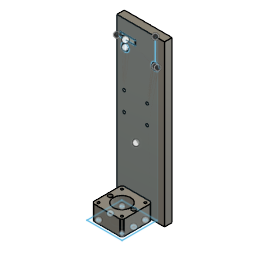
lh_arm_mount_i1 (Autodesk Fusion 360 design; units mm, degrees)
Autodesk Fusion 360 part; units mm, degrees
note: some values were not read from the file. Chosen so that the rebuilt part matches the saved one: which pieces of a blend or face edit are solid.
imported_body "Base Feature1" makes body 1 makes body 2 makes body 3
sketch "Sketch3" plane through (0, 15.85, 0) normal (0, 1, 0) x (-1, 0, 0)
  line L0 (19.8321, 18.0037) -> (18.0037, 19.8321)
  arc A0 (18.0037, 19.8321) -> (17.2966, 20.125) centre (17.2966, 19.125) ccw
  line L1 (17.2966, 20.125) -> (-17.2966, 20.125)
  arc A1 (-17.2966, 20.125) -> (-18.0037, 19.8321) centre (-17.2966, 19.125) ccw
  line L2 (-18.0037, 19.8321) -> (-19.8321, 18.0037)
  arc A2 (-19.8321, 18.0037) -> (-20.125, 17.2966) centre (-19.125, 17.2966) ccw
  line L3 (-20.125, 17.2966) -> (-20.125, -17.2966)
  arc A3 (-20.125, -17.2966) -> (-19.8321, -18.0037) centre (-19.125, -17.2966) ccw
  line L4 (-19.8321, -18.0037) -> (-18.0037, -19.8321)
  arc A4 (-18.0037, -19.8321) -> (-17.2966, -20.125) centre (-17.2966, -19.125) ccw
  line L5 (-17.2966, -20.125) -> (17.2966, -20.125)
  arc A5 (17.2966, -20.125) -> (18.0037, -19.8321) centre (17.2966, -19.125) ccw
  line L6 (18.0037, -19.8321) -> (19.8321, -18.0037)
  arc A6 (19.8321, -18.0037) -> (20.125, -17.2966) centre (19.125, -17.2966) ccw
  line L7 (20.125, -17.2966) -> (20.125, 17.2966)
  arc A7 (20.125, 17.2966) -> (19.8321, 18.0037) centre (19.125, 17.2966) ccw
  circle A8 centre (0, 0) radius 11.5
  line L8 (22.9904, -22.6956) -> (-23.4325, -22.6956)
  line L9 (-23.4325, -22.6956) -> (-23.4325, 23.3044)
  line L10 (-23.4325, 23.3044) -> (22.9904, 23.3044)
  line L11 (22.9904, 23.3044) -> (22.9904, -22.6956)
  circle A9 centre (15.5, 0) radius 2.7
  circle A10 centre (-15.5, 0) radius 2.7
  circle A11 centre (-15.5, 15.5) radius 1.5
  circle A12 centre (15.5, 15.5) radius 1.5
  circle A13 centre (15.5, -15.5) radius 1.5
  circle A14 centre (-15.5, -15.5) radius 1.5
  dimension "d12" = 46
  dimension "d27" = 5.4
  dimension "d28" = 5.4
  dimension "d34" = 3
  dimension "d35" = 3
  dimension "d36" = 3
  dimension "d37" = 3
  constraint horizontal L8
  constraint vertical L9
  constraint horizontal L10
  constraint vertical L11
  measures "d12" distance of L8.start L10.end
  measures "d27" diameter of A9
  measures "d28" diameter of A10
  measures "d34" diameter of A11
  measures "d35" diameter of A12
  measures "d36" diameter of A13
  measures "d37" diameter of A14
extrude "Extrude6" add sketch "Sketch3" along normal blind 20 separate body contours L0 A0 L1 A1 L2 A2 L3 A3 L4 A4 L5 A5 L6 A6 L7 A7 makes body 4
sketch "Sketch5" plane through (0, 0, -20.125) normal (0, 0, -1) x (-1, 0, 0)
  line L0 (-17.2966, 15.85) -> (17.2966, 15.85)
  line L1 (17.2966, 35.85) -> (-17.2966, 35.85)
  line L2 (-27, 227.85) -> (27, 227.85)
  line L3 (27, 227.85) -> (27, 15.85)
  line L4 (27, 15.85) -> (-27, 15.85)
  line L5 (-27, 15.85) -> (-27, 227.85)
  point P0 (0, 15.85)
  dimension "d40" = 54
  dimension "d41" = 212
  constraint horizontal L2
  constraint vertical L3
  constraint horizontal L4
  constraint vertical L5
  constraint midpoint L4 P0
  measures "d40" distance of L2.start L2.end
  measures "d41" distance of L2.start L4.end
extrude "Extrude7" add sketch "Sketch5" along normal blind 10 bodies 4
sketch "Sketch7" plane through (0, 0, -20.125) normal (0, 0, 1) x (1, 0, 0)
  line L0 (17.2966, 35.85) -> (17.2966, 15.85)
  line L1 (17.2966, 15.85) -> (27, 15.85)
  line L2 (27, 15.85) -> (27, 227.85)
  line L3 (27, 227.85) -> (-27, 227.85)
  line L4 (-27, 227.85) -> (-27, 15.85)
  line L5 (-27, 15.85) -> (-17.2966, 15.85)
  line L6 (-17.2966, 15.85) -> (-17.2966, 35.85)
  line L7 (-17.2966, 35.85) -> (17.2966, 35.85)
  line L8 (-17.2966, 35.85) -> (-17.2966, 120.85)
  line L9 (17.2966, 35.85) -> (17.2966, 120.85)
  line L10 (27, 120.85) -> (13.1, 120.85)
  circle A0 centre (13.1, 120.85) radius 1.7
  circle A1 centre (-17.2966, 120.85) radius 1.7
  line L11 (13.1, 120.85) -> (13.1, 145.85)
  line L12 (-17.2966, 120.85) -> (-17.2966, 145.85)
  circle A2 centre (13.1, 145.85) radius 1.7
  circle A3 centre (-17.2966, 145.85) radius 1.7
  dimension "d46" = 85
  dimension "d50" = 85
  dimension "d51" = 13.9
  dimension "d52" = 3.4
  dimension "d54" = 3.4
  dimension "d56" = 25
  dimension "d57" = 25
  dimension "d58" = 3.4
  dimension "d59" = 3.4
  constraint coincident L6.end L7.start
  constraint perpendicular L7 L8
  constraint coincident L0.start L7.end
  constraint perpendicular L7 L9
  constraint coincident L2 L10.start
  constraint perpendicular L2 L10
  constraint coincident L10.end A0.centre
  constraint coincident L8.end A1.centre
  constraint perpendicular L10 L11
  constraint parallel L8 L12
  constraint coincident L11.end A2.centre
  constraint coincident L12.end A3.centre
  measures "d46" distance of L6.end L8.end
  measures "d50" distance of L0.start L9.end
  measures "d51" distance of L10.start L10.end
  measures "d52" diameter of A0
  measures "d54" diameter of A1
  measures "d56" distance of L10.end L11.end
  measures "d57" distance of L8.end L12.end
  measures "d58" diameter of A2
  measures "d59" diameter of A3
hole "Hole2" at (13.1, 120.85, -20.125) at (13.1, 145.85, -20.125) at (-17.2966, 120.85, -20.125) at (-17.2966, 145.85, -20.125) direction (0, 0, -1) diameter 3.4 end through all bodies 4
sketch "Sketch8" plane through (0, 0, -20.125) normal (0, 0, 1) x (1, 0, 0)
  circle A0 centre (-17.2966, 120.85) radius 1.7
  circle A1 centre (13.1, 120.85) radius 1.7
  circle A2 centre (13.1, 145.85) radius 1.7
  circle A3 centre (-17.2966, 145.85) radius 1.7
  line L0 (17.2966, 35.85) -> (17.2966, 15.85)
  line L1 (17.2966, 15.85) -> (27, 15.85)
  line L2 (27, 15.85) -> (27, 227.85)
  line L3 (27, 227.85) -> (-27, 227.85)
  line L4 (-27, 227.85) -> (-27, 15.85)
  line L5 (-27, 15.85) -> (-17.2966, 15.85)
  line L6 (-17.2966, 15.85) -> (-17.2966, 35.85)
  line L7 (-17.2966, 35.85) -> (17.2966, 35.85)
  circle A4 centre (24, 193.8202) radius 4.9
  circle A5 centre (-15.7, 195.8051) radius 4.9
  line L8 (-15.5849, 190.9065) -> (-15.5849, 204.5065)
  line L9 (-27, 204.488) -> (-22, 204.488)
  line L10 (-22, 204.488) -> (-2.4, 204.488)
  line L11 (-2.4, 204.488) -> (-2.4, 210.388)
  line L12 (-2.4, 210.388) -> (-22, 210.388)
  line L13 (-22, 210.388) -> (-22, 204.488)
  line L14 (24, 227.85) -> (24, 193.85)
  line L15 (27, 193.8202) -> (24, 193.8202)
  point P0 (-1.473, 93.6315)
  dimension "d67" = 9.8
  dimension "d70" = 9.8
  dimension "d78" = 13.6
  dimension "d82" = 5
  dimension "d83" = 19.6
  dimension "d84" = 5.9
  dimension "d89" = 34
  dimension "d90" = 3
  constraint coincident A5 L8.start
  constraint coincident L4 L9.start
  constraint perpendicular L4 L9
  constraint horizontal L10
  constraint vertical L11
  constraint horizontal L12
  constraint vertical L13
  constraint coincident L3 L14.start
  constraint perpendicular L3 L14
  constraint coincident L2 L15.start
  constraint perpendicular L2 L15
  constraint coincident A4.centre L15.end
  measures "d67" diameter of A4
  measures "d70" diameter of A5
  measures "d78" distance of L8.start L8.end
  measures "d82" distance of L9.start L9.end
  measures "d83" distance of L9.end L10.end
  measures "d84" distance of L9.end L12.end
  measures "d89" distance of L14.start L14.end
  measures "d90" distance of L15.start A4.centre
hole "Hole3" at (24, 193.85, -20.125) at (-15.7, 195.8051, -20.125) direction (0, 0, -1) diameter 5.4 end through all counterbore diameter 9 counterbore depth 2 bodies 4
extrude "Extrude8" cut sketch "Sketch8" against normal through all contours L10 L11 L12 L13 bodies 4
move_face "OffsetFaces1" offset 9.1 1 faces at (27, 74.0653, -24.125) on bodies 4
hidden bodies 1 2 3
equation "sm_mount_depth = 20 mm"
equation "pipette_plate_width = 54 mm"
equation "pipette_plate_height = 212 mm"
equation "pipette_plate_depth = 10 mm"
equation "sm_mount_width = 46 mm"
equation "d12 = sm_mount_width"
equation "sm_mount_supports_diameter = 3 mm"
equation "d18 = sm_mount_depth"
equation "guide_rod_diameter = 5.4 mm"
equation "d27 = guide_rod_diameter"
equation "d28 = guide_rod_diameter"
equation "d34 = sm_mount_supports_diameter"
equation "d35 = sm_mount_supports_diameter"
equation "d36 = sm_mount_supports_diameter"
equation "d37 = sm_mount_supports_diameter"
equation "d38 = sm_mount_depth"
equation "d40 = pipette_plate_width"
equation "d41 = pipette_plate_height"
equation "d42 = pipette_plate_depth"
equation "d46 = distance_height_pp_holder__scre"
equation "distance_height_pp_holder__scre = 85 mm"
equation "distance_width_pp_holder__scre = 13.9 mm"
equation "d50 = distance_height_pp_holder__scre"
equation "d51 = distance_width_pp_holder__scre"
equation "d52 = m3_diameter"
equation "m3_diameter = 3.4 mm"
equation "d54 = m3_diameter"
equation "distance_between_pp_holder_screws = 25 mm"
equation "d56 = distance_between_pp_holder_screws"
equation "d57 = distance_between_pp_holder_screws"
equation "d58 = m3_diameter"
equation "d59 = m3_diameter"
equation "end3_screw_length_l = 34 mm"
equation "end3_screw_width_l = 12.3 mm"
equation "end3_screw_diameter = 9.8 mm"
equation "d67 = end3_screw_diameter"
equation "d70 = end3_screw_diameter"
equation "end3_screw_outer_circle = 2 mm"
equation "offset_end3_rubber_length = 13.6 mm"
equation "d78 = offset_end3_rubber_length"
equation "offset_end3_rubber_width = 5 mm"
equation "end3_rubber_width = 19.6 mm"
equation "end3_rubber_length = 5.9 mm"
equation "d82 = offset_end3_rubber_width"
equation "d83 = end3_rubber_width"
equation "d84 = end3_rubber_length"
equation "d87 = end3_x_plate_offset"
equation "end3_x_plate_offset = 9.1 mm"
equation "d89 = end3_screw_length_l"
